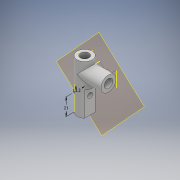
# Autodesk Inventor part: basechassis
Saved by Autodesk Inventor 2018 (Build 220112000, 112)
## iProperties
Created: 2018-11-21
Part Number: basechassis
Material: Generic
Document SubType Name: Modeling
Designer: Prakash
Density: 1 g/cm^3
Appearance: Default
Author: Prakash
Autodesk Inventor part; units mm, degrees
ref_plane "YZ Plane" through (0, 0, 0) normal (1, 0, 0) x (0, 1, 0)
ref_plane "XZ Plane" through (0, 0, 0) normal (0, 1, 0) x (-1, 0, 0)
ref_plane "XY Plane" through (0, 0, 0) normal (0, 0, 1) x (1, 0, 0)
sketch "Sketch1" plane through (0, 0, 0) normal (0, 0, 1) x (1, 0, 0)
  circle A0 centre (0, 0) radius 5.2
  circle A1 centre (0, 0) radius 9.2
  dimension "d0" = 10.4
  dimension "d1" = 18.4
  constraints: 2 centre point, 2 coincident
  measures "d0" diameter of A0
  measures "d1" diameter of A1
extrude "Extrusion1" add sketch "Sketch1" against normal blind 30
sketch "Sketch2" plane through (0, 0, -30) normal (0, 0, -1) x (-1, 0, 0)
  circle A0 centre (0, 0) radius 5.2 projected
  circle A1 centre (0, 0) radius 9.2 projected
  circle A2 centre (0, 0) radius 9.2 projected
  arc A3 (6.5108, 6.5) -> (-6.5108, 6.5) centre (0, 0) ccw
  arc A4 (-6.5108, -6.5) -> (6.5108, -6.5) centre (0, 0) ccw
  line L0 (-6.5108, 6.5) -> (-6.5108, -6.5)
  line L1 (6.5108, 6.5) -> (6.5108, -6.5)
  line L2 (0, 9.2) -> (0, -9.2) construction
  dimension "d4" = 13
  constraints: 12 point on circle, 6 end point, 3 vertical, 2 centre point, 1 midpoint
  measures "d4" distance of L1.start L1.end
extrude "Extrusion2" add sketch "Sketch2" along normal blind 30 contours A0 | L1 A1 L0
ref_plane "Work Plane1" through (9.2, 0, 0) normal (1, 0, 0) x (0, 1, 0)
sketch "Sketch3" plane through (9.2, 0, 0) normal (1, 0, 0) x (0, 1, 0)
  line L0 (9.2, 0) -> (9.2, -60) projected
  line L1 (-9.2, 0) -> (-9.2, -60) projected
  circle A0 centre (0, -15.1245) radius 9.2
  line L2 (9.2, -15.1245) -> (0, -15.1245) construction
  line L3 (0, -15.1245) -> (-9.2, -15.1245) construction
  line L4 (-9.2, 0) -> (9.2, 0) construction
  circle A1 centre (0, -15.1245) radius 5.2
  point P0 (0, 0)
  dimension "d7" = 15.1245
  dimension "d8" = 10.4
  constraints: 4 end point, 3 point on line, 1 centre point, 1 coincident, 1 collinear, 1 horizontal, 1 horizontal alignment, 2 other
  measures "d7" distance from line of L4 L2.end
  measures "d8" diameter of A1
extrude "Extrusion3" add sketch "Sketch3" against normal up to surface contours A0 | A1 round surface about axis through (0, 0, 0) along (0, 0, -1) radius 9.2 far side no
extrude "Extrusion4" add sketch "Sketch3" along normal blind 20
sketch "Sketch4" plane through (-6.5108, -6.5, -30) normal (-1, 0, 0) x (0, 0, 1)
  circle A0 centre (-9, 6.5) radius 6.6
  line L0 (0, 13) -> (0, 0) projected
  line L1 (0, 13) -> (-30, 13) projected
  line L2 (-30, 0) -> (-30, 13) projected
  line L3 (0, 0) -> (-30, 0) projected
  line L4 (-9, 13) -> (-9, 6.5) construction
  line L5 (-9, 6.5) -> (-9, 0) construction
  circle A1 centre (-9, 6.5) radius 3
  point P0 (30, 6.5)
  dimension "d13" = 13.2
  dimension "d14" = 21
  dimension "d15" = 6
  constraints: 4 end point, 3 point on line, 2 centre point, 1 coincident, 1 collinear, 1 vertical
  measures "d13" diameter of A0
  measures "d14" distance from line of L2 L4.end
  measures "d15" diameter of A1
extrude "Extrusion5" cut sketch "Sketch4" against normal blind 5 contours A0 L3 L1 | L1 A0 | A0 L3 | A1
extrude "Extrusion6" cut sketch "Sketch4" against normal up to surface (13.0215 mm away) contours A1
ref_plane "Work Plane3" through (9.2, 9.2, 0) normal (0, 1, 0) x (-1, 0, 0)
sketch "Sketch6" plane through (9.2, 9.2, 0) normal (0, 1, 0) x (-1, 0, 0)
  line L0 (0, -24.3245) -> (9.2, -15.1245) projected
  line L1 (9.2, -15.1245) -> (0, -5.9245) projected
  line L2 (-20, -5.9245) -> (-20, -24.3245) projected
  line L3 (0, -5.9245) -> (-20, -24.3245) construction
  line L4 (0, -24.3245) -> (-20, -5.9245) construction
  point P0 (9.2, 0)
  point P1 (-10, -15.1245)
  constraints: 4 end point, 1 coincident, 1 midpoint
ref_plane "Work Plane4" through (9.2, 9.2, -5.9245) normal (0, -1, 0) x (0.735931, 0, -0.6770565)
sketch "Sketch11" plane through (9.2, 9.2, -5.9245) normal (0, -1, 0) x (0.735931, 0, -0.6770565)
  line L0 (12.4578, -13.5411) -> (14.7186, 13.5411) construction
  line L1 (0, 0) -> (27.1765, 0) construction
  circle A0 centre (13.5882, 0) radius 4
  point P0 (-10.7818, -1.8689)
  dimension "d32" = 8
  constraints: 1 centre point, 1 coincident
  measures "d32" diameter of A0
extrude "Extrusion9" add sketch "Sketch11" along normal up to surface round surface about axis through (9.2, 0, -15.1245) along (-1, 0, 0) radius 9.2 far side no
extrude "Extrusion10" add sketch "Sketch11" against normal blind 1
sketch "Sketch12" plane through (19.2, 10.2, -15.1245) normal (0, 1, 0) x (1, 0, 0)
  line L0 (-10, 9.2) -> (10, -9.2) construction
  line L1 (-10, -9.2) -> (10, 9.2) construction
  circle A0 centre (0, 0) radius 2.5275
  point P0 (-19.2, -15.1245)
  dimension "d37" = 5.055
  constraints: 1 centre point, 1 midpoint
  measures "d37" diameter of A0
extrude "Extrusion11" cut sketch "Sketch12" against normal blind 3.81
sketch "Sketch14" plane through (19.2, 10.2, -15.1245) normal (0, 1, 0) x (1, 0, 0)
  line L0 (-10, -9.2) -> (10, 9.2) construction
  line L1 (-10, 9.2) -> (10, -9.2) construction
  circle A0 centre (0, 0) radius 2.6545
  point P0 (-19.2, -15.1245)
  point P1 (0, 0)
  dimension "d41" = 5.309
  constraints: 1 centre point, 1 coincident
  measures "d41" diameter of A0
loft "Loft2" cut profiles "Sketch14" section 1 edges at (16.6725, 6.39, -15.1245)
sketch "Sketch16" plane through (19.2, 6.39, -15.1245) normal (0, 1, 0) x (1, 0, 0)
  line L0 (-10, 9.2) -> (10, -9.2) construction
  line L1 (-10, -9.2) -> (10, 9.2) construction
  circle A0 centre (0, 0) radius 1.8
  point P0 (-19.2, -15.1245)
  point P1 (0, 0)
  dimension "d47" = 3.6
  constraints: 1 centre point, 1 coincident
  measures "d47" diameter of A0
extrude "Extrusion12" cut sketch "Sketch16" against normal up to surface round surface about axis through (9.2, 0, -15.1245) along (1, 0, 0) radius 5.2 far side no
sketch "Sketch17" plane through (9.2, 9.2, -5.9245) normal (0, -1, 0) x (0.735931, 0, -0.6770565)
  line L0 (12.4578, -13.5411) -> (-0.5416, -12.9995) projected
  line L1 (-0.5416, -12.9995) -> (0, 0) projected
  circle A0 centre (-0.5416, -12.9995) radius 4
  point P0 (-10.7818, -1.8689)
  dimension "d50" = 8
  constraints: 1 centre point, 1 coincident
  measures "d50" diameter of A0
extrude "Extrusion13" add sketch "Sketch17" against normal blind 1
extrude "Extrusion17" add sketch "Sketch17" along normal up to surface round surface about axis through (0, 0, 0) along (0, 0, -1) radius 9.2 far side no
sketch "Sketch21" plane through (0, 10.2, -15.1245) normal (0, 1, 0) x (1, 0, 0)
  line L0 (0, 0) -> (9.2, -9.2) projected
  line L1 (9.2, 9.2) -> (0, 0) projected
  circle A0 centre (0, 0) radius 2.5275
  point P0 (0, -15.1245)
  dimension "d68" = 5.055
  constraints: 1 centre point, 1 coincident
  measures "d68" diameter of A0
extrude "Extrusion18" cut sketch "Sketch21" against normal blind 3.81
sketch "Sketch22" plane through (0, 10.2, -15.1245) normal (0, 1, 0) x (1, 0, 0)
  line L0 (0, 0) -> (9.2, -9.2) projected
  line L1 (9.2, 9.2) -> (0, 0) projected
  circle A0 centre (0, 0) radius 2.6545
  point P0 (0, -15.1245)
  dimension "d71" = 5.309
  constraints: 1 centre point, 1 coincident
  measures "d71" diameter of A0
loft "Loft4" cut profiles "Sketch22" section 1 edges at (-2.5275, 6.39, -15.1245)
sketch "Sketch23" plane through (0, 6.39, -15.1245) normal (0, 1, 0) x (1, 0, 0)
  line L0 (9.2, 9.2) -> (0, 0) projected
  line L1 (0, 0) -> (9.2, -9.2) projected
  circle A0 centre (0, 0) radius 1.8
  point P0 (0, -15.1245)
  dimension "d76" = 3.6
  constraints: 1 centre point, 1 coincident
  measures "d76" diameter of A0
extrude "Extrusion19" cut sketch "Sketch23" against normal up to surface round surface about axis through (0, 0, 0) along (0, 0, -1) radius 5.2 far side no
body "Solid1"
